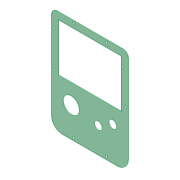
# Autodesk Inventor part: lcd_spacer
Saved by Autodesk Inventor 2014 (Build 180170000, 170)
## iProperties
Created: 2013-06-23
Part Number: lcd_spacer
Document SubType Name: Modeling
Designer: Administrator
Density: 1 g/cm^3
Material: Generic
Appearance: Clear - Green 1
Author: Administrator
Autodesk Inventor part; units mm, degrees
ref_plane "YZ Plane" through (0, 0, 0) normal (1, 0, 0) x (0, 1, 0)
ref_plane "XZ Plane" through (0, 0, 0) normal (0, 1, 0) x (-1, 0, 0)
ref_plane "XY Plane" through (0, 0, 0) normal (0, 0, 1) x (1, 0, 0)
sketch "Sketch1" plane through (0, 0, 0) normal (0, 0, 1) x (1, 0, 0)
  line L0 (11.7695, 33.9618) -> (11.7695, -67.6382)
  line L1 (100.6695, 33.9618) -> (100.6695, -67.6382)
  line L2 (18.1195, 40.3118) -> (94.3195, 40.3118)
  line L3 (24.4695, -80.3382) -> (87.9695, -80.3382)
  arc A0 (11.7695, -67.6382) -> (24.4695, -80.3382) centre (24.4695, -67.6382) ccw
  arc A1 (87.9695, -80.3382) -> (100.6695, -67.6382) centre (87.9695, -67.6382) ccw
  arc A2 (100.6695, 33.9618) -> (94.3195, 40.3118) centre (94.3195, 33.9618) ccw
  arc A3 (18.1195, 40.3118) -> (11.7695, 33.9618) centre (18.1195, 33.9618) ccw
  point P0 (0, 0)
  dimension "d0" = 12.7
  dimension "d1" = 6.35
  dimension "d2" = 120.65
  dimension "d3" = 88.9
  constraints: 8 end point, 8 point on circle, 8 tangent, 4 centre point, 2 equal radius, 2 horizontal, 2 vertical
  measures "d0" radius of A0
  measures "d1" radius of A3
  measures "d2" distance between parallel lines of L3 L2
  measures "d3" distance between parallel lines of L1 L0
extrude "Extrusion1" add sketch "Sketch1" along normal blind 0.7937
sketch "Sketch2" plane through (0, 0, 0.7937) normal (0, 0, 1) x (1, 0, 0)
  line L0 (11.7695, -67.6382) -> (11.7695, 33.9618) projected
  line L1 (100.6695, 33.9618) -> (100.6695, -67.6382) projected
  line L2 (18.1195, 40.3118) -> (94.3195, 40.3118) projected
  line L3 (19.7795, 32.2228) -> (92.6595, 32.2228)
  line L4 (92.6595, 32.2228) -> (92.6595, -23.1372)
  line L5 (92.6595, -23.1372) -> (19.7795, -23.1372)
  line L6 (19.7795, -23.1372) -> (19.7795, 32.2228)
  line L7 (87.9695, -80.3382) -> (24.4695, -80.3382) projected
  point P0 (0, 0)
  dimension "d7" = 8.089
  dimension "d22" = 72.88
  dimension "d23" = 8.01
  dimension "d24" = 8.01
  dimension "d25" = 55.36
  dimension "d70" = 80.89
  dimension "d71" = 57.201
  dimension "d72" = 112.561
  constraints: 8 end point, 2 vertical, 1 horizontal
  measures "d7" distance between parallel lines of L2 L3
  measures "d22" distance of L4.end L5.end
  measures "d23" distance between parallel lines of L0 L6
  measures "d24" distance between parallel lines of L1 L4
  measures "d25" distance of L5.end L3.start
  measures "d70" distance between parallel lines of L0 L4
  measures "d71" distance between parallel lines of L7 L5
  measures "d72" distance between parallel lines of L7 L3
extrude "Extrusion2" cut sketch "Sketch2" against normal through all
sketch "Sketch5" plane through (0, 0, 0.7937) normal (0, 0, 1) x (1, 0, 0)
  circle A0 centre (34.6295, -46.0482) radius 9.398
  circle A1 centre (82.6355, -41.2222) radius 4.572
  circle A2 centre (65.9178, -50.8742) radius 4.572
  line L0 (87.9695, -80.3382) -> (24.4695, -80.3382) projected
  line L1 (11.7695, -67.6382) -> (11.7695, 33.9618) projected
  line L2 (100.6695, 33.9618) -> (100.6695, -67.6382) projected
  line L3 (100.6695, -46.0482) -> (11.7695, -46.0482) construction
  line L4 (65.9178, -50.8742) -> (74.2766, -46.0482) construction
  line L5 (82.6355, -41.2222) -> (74.2766, -46.0482) construction
  line L6 (25.2315, -36.6502) -> (87.2075, -36.6502) construction
  line L7 (87.2075, -36.6502) -> (87.2075, -55.4462) construction
  line L8 (87.2075, -55.4462) -> (25.2315, -55.4462) construction
  line L9 (25.2315, -55.4462) -> (25.2315, -36.6502) construction
  point P0 (0, 0)
  dimension "d26" = 18.796
  dimension "d27" = 9.144
  dimension "d35" = 34.29
  dimension "d40" = 30
  dimension "d41" = 13.462
  dimension "d42" = 13.462
  dimension "d54" = 66.04
  dimension "d55" = 34.7518
  dimension "d56" = 18.034
  dimension "d57" = 29.464
  dimension "d58" = 39.116
  constraints: 14 end point, 6 tangent, 4 point on line, 3 centre point, 3 horizontal, 2 vertical, 1 collinear, 1 equal radius
  measures "d26" diameter of A0
  measures "d27" diameter of A1
  measures "d35" distance between parallel lines of L0 L3
  measures "d40" angle of L3 L4
  measures "d41" distance between parallel lines of L1 L9
  measures "d42" distance between parallel lines of L2 L7
  measures "d54" distance from line of L2 A0.centre
  measures "d55" distance from line of L2 L4.start
  measures "d56" distance from line of L2 L5.start
  measures "d57" distance from line of L0 L4.start
  measures "d58" distance from line of L0 L5.start
extrude "Extrusion5" cut sketch "Sketch5" against normal through all
sketch "Sketch6" plane through (0, 0, 0.7937) normal (0, 0, 1) x (1, 0, 0)
  line L0 (52.111, -71.628) -> (60.3281, -71.628)
  arc A0 (52.111, -71.628) -> (49.1232, -73.533) centre (50.5369, -72.4548) ccw
  arc A1 (49.1232, -73.533) -> (52.111, -75.438) centre (50.5369, -74.6113) ccw
  line L1 (52.111, -75.438) -> (60.3281, -75.438)
  arc A2 (63.3159, -73.533) -> (60.3281, -71.628) centre (61.9022, -72.4548) ccw
  arc A3 (60.3281, -75.438) -> (63.3159, -73.533) centre (61.9022, -74.6113) ccw
  line L2 (11.7695, -67.6382) -> (11.7695, 33.9618) projected
  point P0 (0, 0)
  dimension "d43" = 3.81
  dimension "d44" = 1.778
  dimension "d45" = 8.2171
  dimension "d51" = 40.3415
  dimension "d52" = 2.1565
  constraints: 8 point on circle, 4 centre point, 4 end point, 4 vertical alignment, 3 equal radius, 2 horizontal, 2 horizontal alignment, 1 parallel
  measures "d43" distance between parallel lines of L1 L0
  measures "d44" radius of A0
  measures "d45" distance of L0.start L0.end
  measures "d51" distance from line of L2 L0.start
  measures "d52" distance of A1.centre A0.centre
extrude "Extrusion6" [suppressed]
sketch "Sketch7" plane through (0, 0, 0.7937) normal (0, 0, 1) x (1, 0, 0)
  line L0 (11.7695, -67.6382) -> (11.7695, 33.9618) projected
  line L1 (87.9695, -80.3382) -> (24.4695, -80.3382) projected
  line L2 (100.6695, 33.9618) -> (100.6695, -67.6382) projected
  line L3 (18.1195, 40.3118) -> (94.3195, 40.3118) projected
  circle A0 centre (37.1695, 37.1876) radius 1.27
  circle A1 centre (75.2695, 37.1876) radius 1.27
  circle A2 centre (97.5453, 21.2618) radius 1.27
  circle A3 centre (97.5453, -16.8382) radius 1.27
  circle A4 centre (75.2695, -77.214) radius 1.27
  circle A5 centre (37.1695, -77.214) radius 1.27
  circle A6 centre (14.8937, 21.2618) radius 1.27
  circle A7 centre (14.8937, -16.8382) radius 1.27
  point P0 (0, 0)
  dimension "d59" = 2.54
  dimension "d60" = 3.1242
  dimension "d61" = 3.1242
  dimension "d62" = 3.1242
  dimension "d63" = 3.1242
  dimension "d64" = 25.4
  dimension "d65" = 19.05
  dimension "d66" = 38.1
  dimension "d67" = 38.1
  constraints: 8 centre point, 7 equal radius, 4 horizontal alignment, 4 vertical alignment
  measures "d59" diameter of A0
  measures "d60" distance from line of L0 A6.centre
  measures "d61" distance from line of L2 A2.centre
  measures "d62" distance from line of L3 A1.centre
  measures "d63" distance from line of L1 A5.centre
  measures "d64" distance from line of L0 A0.centre
  measures "d65" distance from line of L3 A6.centre
  measures "d66" distance of A1.centre A0.centre
  measures "d67" distance of A7.centre A6.centre
extrude "Extrusion7" cut sketch "Sketch7" against normal through all
equation "\"d23\" = d24"
equation "\"d42\" = d41"
body "Solid1"
